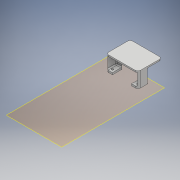
# Autodesk Inventor part: electronics support
Saved by Autodesk Inventor 2017 (Build 210142000, 142)
## iProperties
Created: 2017-07-07
Part Number: electronics support
Material: Generic
Document SubType Name: Modeling
Designer: will
Density: 1 g/cm^3
Appearance: Default
Author: will
Autodesk Inventor part; units mm, degrees
ref_plane "YZ Plane" through (0, 0, 0) normal (1, 0, 0) x (0, 1, 0)
ref_plane "XZ Plane" through (0, 0, 0) normal (0, 1, 0) x (-1, 0, 0)
ref_plane "XY Plane" through (0, 0, 0) normal (0, 0, 1) x (1, 0, 0)
ref_plane "Work Plane1" through (0, 0, 0) normal (0, 0, 1) x (1, 0, 0)
sketch "Sketch1" plane through (0, 0, 0) normal (0, 0, 1) x (1, 0, 0)
  line L0 (-34.9568, 37.8) -> (-33.8, 37.8) projected
  arc A0 (-52.5, 15.282) -> (-34.9568, 37.8) centre (-55.9339, 36.05) ccw projected
  line L1 (-52.5, 15.282) -> (-52.5, -15) projected
  line L2 (-47.7, -15) -> (-52.5, -15) projected
  arc A1 (-33, -29.7) -> (-47.7, -15) centre (-47.7, -29.7) ccw projected
  line L3 (-33, -29.7) -> (-33, -95.5) projected
  arc A2 (-33, -95.5) -> (-31, -97.5) centre (-31, -95.5) ccw projected
  line L4 (-31, -97.5) -> (-22, -97.5) projected
  arc A3 (-22, -97.5) -> (-20, -95.5) centre (-22, -95.5) ccw projected
  line L5 (-20, -74.5) -> (-20, -95.5) projected
  arc A4 (-18, -72.5) -> (-20, -74.5) centre (-18, -74.5) ccw projected
  line L6 (18, -72.5) -> (-18, -72.5) projected
  arc A5 (20, -74.5) -> (18, -72.5) centre (18, -74.5) ccw projected
  line L7 (20, -74.5) -> (20, -95.5) projected
  arc A6 (20, -95.5) -> (22, -97.5) centre (22, -95.5) ccw projected
  line L8 (31, -97.5) -> (22, -97.5) projected
  arc A7 (31, -97.5) -> (33, -95.5) centre (31, -95.5) ccw projected
  line L9 (33, -29.7) -> (33, -95.5) projected
  arc A8 (47.7, -15) -> (33, -29.7) centre (47.7, -29.7) ccw projected
  line L10 (52.5, -15) -> (47.7, -15) projected
  line L11 (52.5, -15) -> (52.5, 15) projected
  line L12 (52.5, 15) -> (47.7, 15) projected
  arc A9 (33, 29.7) -> (47.7, 15) centre (47.7, 29.7) ccw projected
  line L13 (33, 29.7) -> (33, 95.5) projected
  arc A10 (33, 95.5) -> (31, 97.5) centre (31, 95.5) ccw projected
  line L14 (31, 97.5) -> (22, 97.5) projected
  arc A11 (22, 97.5) -> (20, 95.5) centre (22, 95.5) ccw projected
  line L15 (20, 95.5) -> (20, 74.5) projected
  arc A12 (18, 72.5) -> (20, 74.5) centre (18, 74.5) ccw projected
  line L16 (18, 72.5) -> (-18, 72.5) projected
  arc A13 (-20, 74.5) -> (-18, 72.5) centre (-18, 74.5) ccw projected
  line L17 (-20, 74.5) -> (-20, 95.5) projected
  arc A14 (-20, 95.5) -> (-22, 97.5) centre (-22, 95.5) ccw projected
  line L18 (-22, 97.5) -> (-31, 97.5) projected
  arc A15 (-31, 97.5) -> (-33, 95.5) centre (-31, 95.5) ccw projected
  line L19 (-33, 95.5) -> (-33, 74.5) projected
  arc A16 (-33.8, 72.9) -> (-33, 74.5) centre (-35, 74.5) ccw projected
  line L20 (-33.8, 72.9) -> (-33.8, 37.8) projected
  circle A17 centre (-21.8, 62.5) radius 3 projected
  circle A18 centre (26.5, 62.5) radius 4 projected
  arc A19 (-2.5981, -57.75) -> (2.5981, -57.75) centre (0, -56.25) ccw projected
  line L21 (-2.5981, -57.75) -> (-13, -57.75) projected
  line L22 (-13, -57.75) -> (-13, -54.75) projected
  line L23 (-2.5981, -54.75) -> (-13, -54.75) projected
  arc A20 (2.5981, -54.75) -> (-2.5981, -54.75) centre (0, -56.25) ccw projected
  line L24 (13, -54.75) -> (2.5981, -54.75) projected
  line L25 (13, -57.75) -> (13, -54.75) projected
  line L26 (13, -57.75) -> (2.5981, -57.75) projected
  circle A21 centre (-10.5, -67.75) radius 1.5 projected
  circle A22 centre (10.5, -67.75) radius 1.5 projected
  line L27 (-19.3171, -45) -> (-23.6904, -45) projected
  line L28 (-23.6904, -45) -> (-23.6904, -25.95) projected
  line L29 (-23.6904, -25.95) -> (-19.382, -25.95) projected
  spline S0 degree 3 poles (-19.382, -25.95) (-19.0461, -25.9523) (-18.3968, -25.9567) (-17.4563, -26.0086) (-16.581, -26.0848) (-15.773, -26.2013) (-15.0294, -26.3366) (-14.3557, -26.5178) (-13.7463, -26.7258) (-13.195, -26.968) (-12.693, -27.2522) (-12.2198, -27.5714) (-11.7698, -27.9304) (-11.3405, -28.3302) (-10.931, -28.768) (-10.5507, -29.2527) (-10.1877, -29.7717) (-9.8476, -30.3268) (-9.5449, -30.9169) (-9.2755, -31.5328) (-9.051, -32.1747) (-8.8682, -32.8419) (-8.7226, -33.5324) (-8.6207, -34.2476) (-8.5577, -34.9867) (-8.5513, -35.4876) (-8.5481, -35.7421) knots 0 0 0 0 0.060145 0.116262 0.168646 0.217421 0.26241 0.303907 0.342233 0.377621 0.411584 0.445386 0.479752 0.514569 0.550351 0.586994 0.624785 0.663736 0.70347 0.743462 0.784023 0.82514 0.867271 0.910311 0.954426 1 1 1 1 projected
  spline S1 degree 3 poles (-8.5481, -35.7421) (-8.5566, -36.1013) (-8.5733, -36.8083) (-8.7143, -37.8459) (-8.9423, -38.8405) (-9.263, -39.7843) (-9.6601, -40.6693) (-10.1357, -41.4778) (-10.6762, -42.2113) (-11.2862, -42.8578) (-11.9457, -43.4169) (-12.6337, -43.8901) (-13.3497, -44.2699) (-13.9819, -44.5071) (-14.5316, -44.6562) (-15.0135, -44.7428) (-15.562, -44.8231) (-16.1791, -44.8922) (-16.8667, -44.9395) (-17.6225, -44.9721) (-18.4469, -44.9964) (-19.0195, -44.9988) (-19.3171, -45) knots 0 0 0 0 0.065767 0.129467 0.191414 0.252424 0.311761 0.368786 0.423917 0.478313 0.53121 0.582008 0.630995 0.679292 0.705349 0.735235 0.768913 0.806892 0.848943 0.895126 0.945474 1 1 1 1 projected
  line L30 (3.7964, 45) -> (7.4446, 45) projected
  line L31 (7.4446, 45) -> (-0.2525, 25.95) projected
  line L32 (-0.2525, 25.95) -> (-3.4237, 25.95) projected
  line L33 (-3.4237, 25.95) -> (-11.1169, 45) projected
  line L34 (-11.1169, 45) -> (-7.4649, 45) projected
  line L35 (-7.4649, 45) -> (-5.9843, 41.0923) projected
  line L36 (-5.9843, 41.0923) -> (2.3158, 41.0923) projected
  line L37 (2.3158, 41.0923) -> (3.7964, 45) projected
  spline S2 degree 3 poles (-13.4371, 30.2927) (-13.4413, 30.1296) (-13.4494, 29.8083) (-13.522, 29.3359) (-13.6305, 28.88) (-13.7882, 28.4424) (-13.9927, 28.0235) (-14.2412, 27.6214) (-14.5373, 27.2397) (-14.8711, 26.8787) (-15.2388, 26.5488) (-15.6318, 26.2577) (-16.0477, 26.0117) (-16.4842, 25.8077) (-16.9438, 25.6516) (-17.4232, 25.5409) (-17.923, 25.475) (-18.263, 25.4661) (-18.4362, 25.4615) knots 0 0 0 0 0.063173 0.124457 0.184841 0.244567 0.304319 0.3652 0.427421 0.491262 0.555499 0.618605 0.680495 0.742473 0.804991 0.868252 0.932887 1 1 1 1 projected
  spline S3 degree 3 poles (-18.4362, 25.4615) (-18.6607, 25.4697) (-19.1078, 25.4861) (-19.7689, 25.614) (-20.4146, 25.8152) (-20.935, 26.0578) (-21.349, 26.2929) (-21.6663, 26.5093) (-21.9892, 26.7572) (-22.3203, 27.0374) (-22.6533, 27.3552) (-22.9979, 27.703) (-23.3493, 28.0837) (-23.5776, 28.3557) (-23.6948, 28.4953) knots 0 0 0 0 0.10691 0.212977 0.319777 0.428556 0.485857 0.546559 0.611431 0.679821 0.753159 0.830753 0.913133 1 1 1 1 projected
  line L38 (-23.6948, 28.4953) -> (-21.138, 30.8346) projected
  spline S4 degree 3 poles (-21.138, 30.8346) (-21.0285, 30.6801) (-20.8182, 30.3835) (-20.4774, 29.9864) (-20.1381, 29.6476) (-19.7972, 29.3685) (-19.4517, 29.1509) (-19.1022, 28.9969) (-18.7506, 28.899) (-18.5144, 28.8868) (-18.3981, 28.8808) knots 0 0 0 0 0.16242 0.311824 0.448433 0.573381 0.689077 0.797573 0.900293 1 1 1 1 projected
  spline S5 degree 3 poles (-18.3981, 28.8808) (-18.2895, 28.8846) (-18.08, 28.8919) (-17.7813, 28.965) (-17.5161, 29.091) (-17.2847, 29.2559) (-17.1014, 29.4544) (-16.955, 29.6627) (-16.8726, 29.8926) (-16.8617, 30.0505) (-16.8564, 30.1286) knots 0 0 0 0 0.148126 0.285993 0.416634 0.54738 0.671583 0.784401 0.893266 1 1 1 1 projected
  spline S6 degree 3 poles (-16.8564, 30.1286) (-16.8597, 30.2079) (-16.8665, 30.3676) (-16.932, 30.6016) (-17.0306, 30.8303) (-17.1249, 30.9695) (-17.1731, 31.0407) knots 0 0 0 0 0.241881 0.487115 0.737838 1 1 1 1 projected
  spline S7 degree 3 poles (-17.1731, 31.0407) (-17.2169, 31.096) (-17.3177, 31.2233) (-17.51, 31.425) (-17.7515, 31.672) (-18.0515, 31.9559) (-18.3975, 32.2869) (-18.8055, 32.6521) (-19.2639, 33.0626) (-19.5897, 33.3485) (-19.7604, 33.4983) knots 0 0 0 0 0.059234 0.136349 0.233805 0.349411 0.483179 0.635967 0.809243 1 1 1 1 projected
  spline S8 degree 3 poles (-19.7604, 33.4983) (-19.9207, 33.6369) (-20.2248, 33.9001) (-20.6575, 34.2737) (-21.0377, 34.6098) (-21.3711, 34.9034) (-21.6525, 35.1575) (-21.8832, 35.3734) (-22.066, 35.5468) (-22.1698, 35.6516) (-22.2142, 35.6963) knots 0 0 0 0 0.192953 0.366184 0.520457 0.655012 0.770624 0.865677 0.942675 1 1 1 1 projected
  spline S9 degree 3 poles (-22.2142, 35.6963) (-22.3823, 35.8783) (-22.7056, 36.2282) (-23.1258, 36.7704) (-23.4717, 37.2997) (-23.7392, 37.8261) (-23.9412, 38.3571) (-24.0837, 38.9058) (-24.169, 39.4779) (-24.1785, 39.8683) (-24.1833, 40.0658) knots 0 0 0 0 0.150833 0.289954 0.417139 0.535255 0.648751 0.762405 0.879827 1 1 1 1 projected
  spline S10 degree 3 poles (-24.1833, 40.0658) (-24.1799, 40.2582) (-24.1732, 40.6357) (-24.0912, 41.1881) (-23.9744, 41.7167) (-23.7937, 42.2159) (-23.5735, 42.6938) (-23.2975, 43.143) (-22.9733, 43.568) (-22.6017, 43.9612) (-22.1907, 44.318) (-21.7499, 44.6356) (-21.2749, 44.8978) (-20.7698, 45.1138) (-20.2349, 45.2801) (-19.6709, 45.403) (-19.0767, 45.4768) (-18.6705, 45.4845) (-18.4629, 45.4885) knots 0 0 0 0 0.065201 0.127927 0.189047 0.248544 0.307607 0.367248 0.426963 0.488617 0.550392 0.611331 0.672556 0.734024 0.797341 0.86225 0.929625 1 1 1 1 projected
  spline S11 degree 3 poles (-18.4629, 45.4885) (-18.3, 45.4856) (-17.9773, 45.4798) (-17.5017, 45.4331) (-17.0425, 45.3577) (-16.6001, 45.2496) (-16.1726, 45.1126) (-15.76, 44.9452) (-15.3651, 44.745) (-14.9849, 44.5159) (-14.6212, 44.2499) (-14.2696, 43.9524) (-13.9334, 43.6189) (-13.611, 43.2501) (-13.3046, 42.8451) (-13.004, 42.4093) (-12.7227, 41.9348) (-12.549, 41.602) (-12.4602, 41.4319) knots 0 0 0 0 0.063551 0.125868 0.18624 0.244977 0.303358 0.36123 0.418489 0.475937 0.534204 0.594059 0.655469 0.718772 0.784975 0.853522 0.925182 1 1 1 1 projected
  line L39 (-12.4602, 41.4319) -> (-15.4673, 39.6269) projected
  spline S12 degree 3 poles (-15.4673, 39.6269) (-15.5783, 39.8199) (-15.7912, 40.1899) (-16.1519, 40.687) (-16.5214, 41.1127) (-16.9082, 41.4595) (-17.3078, 41.7319) (-17.7219, 41.9266) (-18.1509, 42.0472) (-18.4431, 42.0619) (-18.5889, 42.0692) knots 0 0 0 0 0.160458 0.307612 0.442139 0.566229 0.681222 0.789558 0.895029 1 1 1 1 projected
  spline S13 degree 3 poles (-18.5889, 42.0692) (-18.7371, 42.0632) (-19.0248, 42.0516) (-19.4353, 41.9442) (-19.8118, 41.7754) (-20.1371, 41.5347) (-20.4127, 41.2569) (-20.616, 40.9478) (-20.7437, 40.6134) (-20.7572, 40.3811) (-20.764, 40.2642) knots 0 0 0 0 0.141986 0.275473 0.404346 0.53543 0.661427 0.777867 0.88828 1 1 1 1 projected
  spline S14 degree 3 poles (-20.764, 40.2642) (-20.7578, 40.1555) (-20.745, 39.9347) (-20.6512, 39.6064) (-20.5044, 39.2782) (-20.3309, 39.009) (-20.1542, 38.7836) (-19.9853, 38.5884) (-19.7796, 38.3726) (-19.5377, 38.1361) (-19.2627, 37.8768) (-18.9544, 37.5947) (-18.6093, 37.2923) (-18.3653, 37.0863) (-18.2378, 36.9785) knots 0 0 0 0 0.076347 0.155091 0.238352 0.328404 0.379384 0.439618 0.509831 0.588875 0.677436 0.775547 0.882636 1 1 1 1 projected
  spline S15 degree 3 poles (-18.2378, 36.9785) (-17.9953, 36.7734) (-17.5299, 36.3796) (-16.8723, 35.7981) (-16.2797, 35.2545) (-15.7573, 34.7423) (-15.2983, 34.2709) (-14.906, 33.8364) (-14.5847, 33.4355) (-14.2465, 32.9607) (-13.9251, 32.3821) (-13.6474, 31.686) (-13.4672, 30.99) (-13.4471, 30.5227) (-13.4371, 30.2927) knots 0 0 0 0 0.112125 0.215201 0.309902 0.395959 0.473447 0.54214 0.602523 0.654726 0.747804 0.835278 0.918925 1 1 1 1 projected
  spline S16 degree 3 poles (13.9212, -30.2927) (13.9253, -30.1296) (13.9334, -29.8083) (14.006, -29.3358) (14.1149, -28.8801) (14.2713, -28.4413) (14.4812, -28.0244) (14.7291, -27.6225) (15.0221, -27.237) (15.3579, -26.8764) (15.7266, -26.5449) (16.1197, -26.2541) (16.5338, -26.0081) (16.9701, -25.8078) (17.4277, -25.6514) (17.9072, -25.5409) (18.4071, -25.475) (18.7471, -25.4661) (18.9203, -25.4615) knots 0 0 0 0 0.063175 0.124462 0.184848 0.244577 0.304549 0.365432 0.427356 0.491896 0.556136 0.619244 0.681136 0.742463 0.804983 0.868247 0.932885 1 1 1 1 projected
  spline S17 degree 3 poles (18.9203, -25.4615) (19.1447, -25.4698) (19.5918, -25.4862) (20.2531, -25.6138) (20.8993, -25.8165) (21.4216, -26.0553) (21.8337, -26.2941) (22.1502, -26.5094) (22.4748, -26.7567) (22.8016, -27.0431) (23.1428, -27.3521) (23.4813, -27.7049) (23.8337, -28.0834) (24.0618, -28.3556) (24.1788, -28.4953) knots 0 0 0 0 0.106908 0.212971 0.319769 0.429097 0.485871 0.546571 0.611442 0.680224 0.75359 0.830757 0.913135 1 1 1 1 projected
  line L40 (24.1788, -28.4953) -> (21.6221, -30.8346) projected
  spline S18 degree 3 poles (21.6221, -30.8346) (21.5126, -30.6801) (21.3023, -30.3834) (20.9612, -29.9866) (20.6222, -29.6459) (20.2782, -29.371) (19.9353, -29.1497) (19.5861, -28.9971) (19.2347, -28.8989) (18.9984, -28.8868) (18.8821, -28.8808) knots 0 0 0 0 0.162432 0.311848 0.448466 0.574275 0.689054 0.797558 0.900286 1 1 1 1 projected
  spline S19 degree 3 poles (18.8821, -28.8808) (18.7735, -28.8845) (18.5639, -28.8916) (18.2664, -28.966) (17.9991, -29.0863) (17.769, -29.2525) (17.584, -29.4509) (17.4401, -29.6621) (17.3564, -29.8925) (17.3457, -30.0504) (17.3404, -30.1286) knots 0 0 0 0 0.14802 0.285787 0.415605 0.546256 0.67037 0.784556 0.893342 1 1 1 1 projected
  spline S20 degree 3 poles (17.3404, -30.1286) (17.3437, -30.2079) (17.3505, -30.3676) (17.416, -30.6016) (17.5147, -30.8303) (17.6089, -30.9695) (17.6571, -31.0407) knots 0 0 0 0 0.241881 0.487115 0.737838 1 1 1 1 projected
  spline S21 degree 3 poles (17.6571, -31.0407) (17.7011, -31.0958) (17.8029, -31.2235) (17.9912, -31.4289) (18.2374, -31.6701) (18.5311, -31.9592) (18.8833, -32.2849) (19.2865, -32.6567) (19.7496, -33.0619) (20.0741, -33.348) (20.2444, -33.4983) knots 0 0 0 0 0.059231 0.13713 0.233823 0.348656 0.483195 0.636695 0.809253 1 1 1 1 projected
  spline S22 degree 3 poles (20.2444, -33.4983) (20.4047, -33.6369) (20.7089, -33.9) (21.1411, -34.2741) (21.5235, -34.6091) (21.8525, -34.9076) (22.1379, -35.1573) (22.3671, -35.3735) (22.55, -35.5468) (22.6539, -35.6516) (22.6982, -35.6963) knots 0 0 0 0 0.192953 0.366186 0.520459 0.655785 0.770623 0.865677 0.942674 1 1 1 1 projected
  spline S23 degree 3 poles (22.6982, -35.6963) (22.8665, -35.8783) (23.1899, -36.2281) (23.6095, -36.7716) (23.9585, -37.298) (24.2288, -37.8224) (24.4248, -38.3553) (24.5675, -38.9046) (24.6531, -39.4779) (24.6625, -39.8683) (24.6673, -40.0658) knots 0 0 0 0 0.150802 0.289894 0.417473 0.534875 0.648075 0.762455 0.879852 1 1 1 1 projected
  spline S24 degree 3 poles (24.6673, -40.0658) (24.6639, -40.2582) (24.6572, -40.6357) (24.5753, -41.1881) (24.4583, -41.7167) (24.2781, -42.2161) (24.0566, -42.6924) (23.7866, -43.1456) (23.4565, -43.5652) (23.0899, -43.9625) (22.678, -44.3191) (22.2351, -44.6335) (21.7603, -44.899) (21.2573, -45.1177) (20.7198, -45.2801) (20.1561, -45.4028) (19.5608, -45.4768) (19.1545, -45.4845) (18.947, -45.4885) knots 0 0 0 0 0.06519 0.127905 0.189015 0.248502 0.307556 0.366963 0.426931 0.48828 0.550044 0.611324 0.672163 0.734187 0.796953 0.862273 0.929637 1 1 1 1 projected
  spline S25 degree 3 poles (18.947, -45.4885) (18.784, -45.4856) (18.4613, -45.4799) (17.9858, -45.4331) (17.5265, -45.3578) (17.0843, -45.2491) (16.6566, -45.1145) (16.2479, -44.9395) (15.8528, -44.7415) (15.4726, -44.5122) (15.1104, -44.2458) (14.7559, -43.9529) (14.4216, -43.6174) (14.0947, -43.2516) (13.7889, -42.8448) (13.488, -42.4094) (13.2068, -41.9348) (13.033, -41.602) (12.9442, -41.4319) knots 0 0 0 0 0.063568 0.125901 0.186289 0.24504 0.303437 0.361056 0.418329 0.475792 0.534074 0.593626 0.655051 0.718698 0.784919 0.853484 0.925163 1 1 1 1 projected
  line L41 (12.9442, -41.4319) -> (15.9513, -39.6269) projected
  spline S26 degree 3 poles (15.9513, -39.6269) (16.0623, -39.8199) (16.2752, -40.1899) (16.6359, -40.687) (17.0054, -41.1127) (17.3923, -41.4595) (17.7918, -41.7319) (18.2059, -41.9266) (18.6349, -42.0472) (18.9271, -42.0619) (19.0729, -42.0692) knots 0 0 0 0 0.160458 0.307612 0.442139 0.566229 0.681222 0.789558 0.895029 1 1 1 1 projected
  spline S27 degree 3 poles (19.0729, -42.0692) (19.2212, -42.0633) (19.5089, -42.0518) (19.9202, -41.9432) (20.299, -41.7767) (20.6246, -41.5344) (20.9012, -41.2581) (21.0994, -40.9466) (21.228, -40.6135) (21.2414, -40.3811) (21.2481, -40.2642) knots 0 0 0 0 0.141922 0.275349 0.405274 0.536299 0.66224 0.777967 0.88833 1 1 1 1 projected
  spline S28 degree 3 poles (21.2481, -40.2642) (21.2418, -40.1555) (21.229, -39.9347) (21.1354, -39.6062) (20.9879, -39.2793) (20.8186, -39.0084) (20.642, -38.7825) (20.469, -38.5898) (20.2639, -38.3723) (20.0216, -38.1362) (19.7467, -37.8768) (19.4384, -37.5947) (19.0933, -37.2923) (18.8494, -37.0863) (18.7218, -36.9785) knots 0 0 0 0 0.076338 0.155074 0.238325 0.327891 0.378865 0.43968 0.509886 0.588921 0.677472 0.775572 0.882649 1 1 1 1 projected
  spline S29 degree 3 poles (18.7218, -36.9785) (18.4793, -36.7734) (18.014, -36.3796) (17.3562, -35.7981) (16.764, -35.2543) (16.2411, -34.7437) (15.7861, -34.2697) (15.394, -33.8364) (15.0711, -33.4353) (14.7362, -32.9562) (14.4091, -32.3806) (14.131, -31.6849) (13.9513, -30.99) (13.9311, -30.5227) (13.9212, -30.2927) knots 0 0 0 0 0.11214 0.215231 0.309946 0.396015 0.473203 0.541905 0.602297 0.654875 0.748186 0.835255 0.918914 1 1 1 1 projected
  line L42 (-3.3124, -45) -> (-6.9606, -45) projected
  line L43 (-6.9606, -45) -> (0.7365, -25.95) projected
  line L44 (0.7365, -25.95) -> (3.9077, -25.95) projected
  line L45 (3.9077, -25.95) -> (11.601, -45) projected
  line L46 (11.601, -45) -> (7.9489, -45) projected
  line L47 (7.9489, -45) -> (6.4683, -41.0923) projected
  line L48 (6.4683, -41.0923) -> (-1.8317, -41.0923) projected
  line L49 (-1.8317, -41.0923) -> (-3.3124, -45) projected
  line L50 (19.8012, 45) -> (24.1744, 45) projected
  line L51 (24.1744, 45) -> (24.1744, 25.95) projected
  line L52 (24.1744, 25.95) -> (19.866, 25.95) projected
  spline S30 degree 3 poles (19.866, 25.95) (19.5301, 25.9523) (18.8809, 25.9569) (17.9402, 26.008) (17.0655, 26.0867) (16.2562, 26.1949) (15.514, 26.338) (14.8397, 26.5176) (14.2313, 26.7249) (13.6819, 26.9689) (13.1804, 27.2533) (12.7041, 27.57) (12.2542, 27.9308) (11.8241, 28.3287) (11.4196, 28.7709) (11.0337, 29.25) (10.6761, 29.7731) (10.3359, 30.3276) (10.0282, 30.9159) (9.7598, 31.5329) (9.5349, 32.1747) (9.3523, 32.8419) (9.2066, 33.5324) (9.1047, 34.2476) (9.0417, 34.9867) (9.0354, 35.4876) (9.0321, 35.7421) knots 0 0 0 0 0.060148 0.116267 0.168654 0.217399 0.262434 0.303933 0.34226 0.377441 0.411406 0.445398 0.479766 0.514584 0.550214 0.587001 0.624663 0.663615 0.703456 0.74345 0.784013 0.825133 0.867265 0.910306 0.954424 1 1 1 1 projected
  spline S31 degree 3 poles (9.0321, 35.7421) (9.0406, 36.1013) (9.0573, 36.8083) (9.1983, 37.8459) (9.4263, 38.8405) (9.7469, 39.7844) (10.1444, 40.6691) (10.6192, 41.4791) (11.1644, 42.21) (11.7737, 42.8582) (12.4333, 43.4153) (13.1189, 43.8925) (13.8369, 44.2687) (14.4696, 44.5073) (15.0183, 44.6557) (15.5, 44.7434) (16.0471, 44.8238) (16.6649, 44.886) (17.3504, 44.9414) (18.1066, 44.9715) (18.9309, 44.9965) (19.5035, 44.9988) (19.8012, 45) knots 0 0 0 0 0.065773 0.129478 0.19143 0.252446 0.311787 0.368818 0.424092 0.478492 0.531394 0.582004 0.631201 0.679503 0.705561 0.735222 0.769132 0.806858 0.84893 0.895117 0.94547 1 1 1 1 projected
  line L53 (33, 76.3047) -> (-33, 76.3047)
  line L54 (20, 76.3047) -> (33, 76.3047)
  line L55 (-33, 76.3047) -> (-20, 76.3047)
  point P0 (0, 0)
  constraints: 6 end point, 6 point on line, 1 collinear, 1 perpendicular
extrude "Extrusion1" add sketch "Sketch1" along normal blind 4 contours L19 A15 L18 A14 L17 L53 | L15 A11 L14 A10 L13 L53
sketch "Sketch2" plane through (0, 0, 4) normal (0, 0, 1) x (1, 0, 0)
  arc A0 (33, 95.5) -> (31, 97.5) centre (31, 95.5) ccw projected
  line L0 (31, 97.5) -> (22, 97.5) projected
  arc A1 (22, 97.5) -> (20, 95.5) centre (22, 95.5) ccw projected
  line L1 (20, 95.5) -> (20, 76.3047) projected
  line L2 (20, 76.3047) -> (33, 76.3047) projected
  line L3 (33, 76.3047) -> (33, 95.5) projected
  arc A2 (-20, 95.5) -> (-22, 97.5) centre (-22, 95.5) ccw projected
  line L4 (-22, 97.5) -> (-31, 97.5) projected
  arc A3 (-31, 97.5) -> (-33, 95.5) centre (-31, 95.5) ccw projected
  line L5 (-33, 95.5) -> (-33, 76.3047) projected
  line L6 (-33, 76.3047) -> (-20, 76.3047) projected
  line L7 (-20, 76.3047) -> (-20, 95.5) projected
  circle A4 centre (27, 82.3047) radius 2
  circle A5 centre (-26, 82.3047) radius 2
  point P0 (0, 0)
  dimension "d2" = 6
  dimension "d3" = 6
  dimension "d4" = 6
  dimension "d5" = 6
  dimension "d6" = 4
  dimension "d7" = 4
  constraints: 2 centre point
  measures "d2" distance from line of L3 A4.centre
  measures "d3" distance from line of L2 A4.centre
  measures "d4" distance from line of L7 A5.centre
  measures "d5" distance from line of L6 A5.centre
  measures "d6" diameter of A4
  measures "d7" diameter of A5
extrude "Extrusion2" cut sketch "Sketch2" against normal blind 7 contours A4 | A5
sketch "Sketch3" plane through (0, 0, 4) normal (0, 0, 1) x (1, 0, 0)
  circle A0 centre (27, 82.3047) radius 2 projected
  arc A1 (33, 95.5) -> (31, 97.5) centre (31, 95.5) ccw projected
  line L0 (31, 97.5) -> (22, 97.5) projected
  arc A2 (22, 97.5) -> (20, 95.5) centre (22, 95.5) ccw projected
  line L1 (20, 95.5) -> (20, 76.3047) projected
  line L2 (20, 76.3047) -> (33, 76.3047) projected
  line L3 (33, 76.3047) -> (33, 95.5) projected
  circle A3 centre (-26, 82.3047) radius 2 projected
  arc A4 (-20, 95.5) -> (-22, 97.5) centre (-22, 95.5) ccw projected
  line L4 (-22, 97.5) -> (-31, 97.5) projected
  arc A5 (-31, 97.5) -> (-33, 95.5) centre (-31, 95.5) ccw projected
  line L5 (-33, 95.5) -> (-33, 76.3047) projected
  line L6 (-33, 76.3047) -> (-20, 76.3047) projected
  line L7 (-20, 76.3047) -> (-20, 95.5) projected
  line L8 (20, 76.3047) -> (33, 76.3047) projected
  line L9 (-33, 76.3047) -> (-20, 76.3047) projected
  line L10 (-31, 76.3047) -> (-31, 95.5)
  line L11 (-31, 95.5) -> (-22, 95.5)
  line L12 (-22, 95.5) -> (-20, 95.5)
  line L13 (31, 76.3047) -> (31, 95.5)
  line L14 (31, 95.5) -> (22, 95.5)
  line L15 (22, 95.5) -> (20, 95.5)
  line L16 (-33, 95.5) -> (-33, 76.3047) projected
  line L17 (-31, 76.3047) -> (-33, 76.3047)
  line L18 (-33, 76.3047) -> (-33, 95.5)
  line L19 (-20, 76.3047) -> (-20, 95.5) projected
  line L20 (-20, 95.5) -> (-20, 76.3047)
  line L21 (-20, 76.3047) -> (-31, 76.3047)
  arc A6 (22, 97.5) -> (20, 95.5) centre (22, 95.5) ccw projected
  line L22 (20, 95.5) -> (20, 76.3047)
  line L23 (20, 76.3047) -> (31, 76.3047)
  point P0 (0, 0)
  constraints: 24 end point, 6 collinear, 4 perpendicular, 2 point on line, 1 horizontal, 1 tangent, 1 vertical
extrude "Extrusion3" add sketch "Sketch3" along normal blind 25 contours L3 L2 L13 L14 L15 A2 L0 A1 | L12 L11 L10 L6 L5 A5 L4 A4
fillet "Fillet1" radius 2 6 edges at (31, 95.5, 16.5) (-31, 95.5, 16.5) (-25.5, 95.5, 4) (-31, 85.9023, 4) (25.5, 95.5, 4) (31, 85.9023, 4)
sketch "Sketch4" plane through (0, 0, 29) normal (0, 0, 1) x (1, 0, 0)
  arc A0 (33, 95.5) -> (31, 97.5) centre (31, 95.5) ccw projected
  line L0 (31, 97.5) -> (22, 97.5) projected
  arc A1 (22, 97.5) -> (20, 95.5) centre (22, 95.5) ccw projected
  line L1 (20, 95.5) -> (29, 95.5) projected
  arc A2 (31, 93.5) -> (29, 95.5) centre (29, 93.5) ccw projected
  line L2 (31, 93.5) -> (31, 76.3047) projected
  line L3 (31, 76.3047) -> (33, 76.3047) projected
  line L4 (33, 76.3047) -> (33, 95.5) projected
  arc A3 (-20, 95.5) -> (-22, 97.5) centre (-22, 95.5) ccw projected
  line L5 (-22, 97.5) -> (-31, 97.5) projected
  arc A4 (-31, 97.5) -> (-33, 95.5) centre (-31, 95.5) ccw projected
  line L6 (-33, 95.5) -> (-33, 76.3047) projected
  line L7 (-33, 76.3047) -> (-31, 76.3047) projected
  line L8 (-31, 76.3047) -> (-31, 93.5) projected
  arc A5 (-29, 95.5) -> (-31, 93.5) centre (-29, 93.5) ccw projected
  line L9 (-29, 95.5) -> (-20, 95.5) projected
  line L10 (33, 76.3047) -> (-33, 76.3047)
  line L11 (-33, 76.3047) -> (-33, 126.3047)
  line L12 (-33, 126.3047) -> (33, 126.3047)
  line L13 (33, 126.3047) -> (33, 76.3047)
  point P0 (0, 0)
  dimension "d13" = 50
  constraints: 8 end point, 2 parallel, 1 horizontal, 1 perpendicular
  measures "d13" distance of L10.end L11.end
extrude "Extrusion4" add sketch "Sketch4" along normal blind 3
fillet "Fillet2" radius 2 6 edges at (26.5, 97.5, 29) (32.4142, 96.9142, 29) (20.5858, 96.9142, 29) (-32.4142, 96.9142, 29) (-20.5858, 96.9142, 29) (-26.5, 97.5, 29)
fillet "Fillet3" radius 5.5 4 edges at (-33, 126.3047, 30.5) (33, 126.3047, 30.5) (-33, 76.3047, 16) (33, 76.3047, 16)
equation "\"d4\" = d2"
equation "\"d5\" = d3"
equation "\"d7\" = d6"
body "Solid1"
